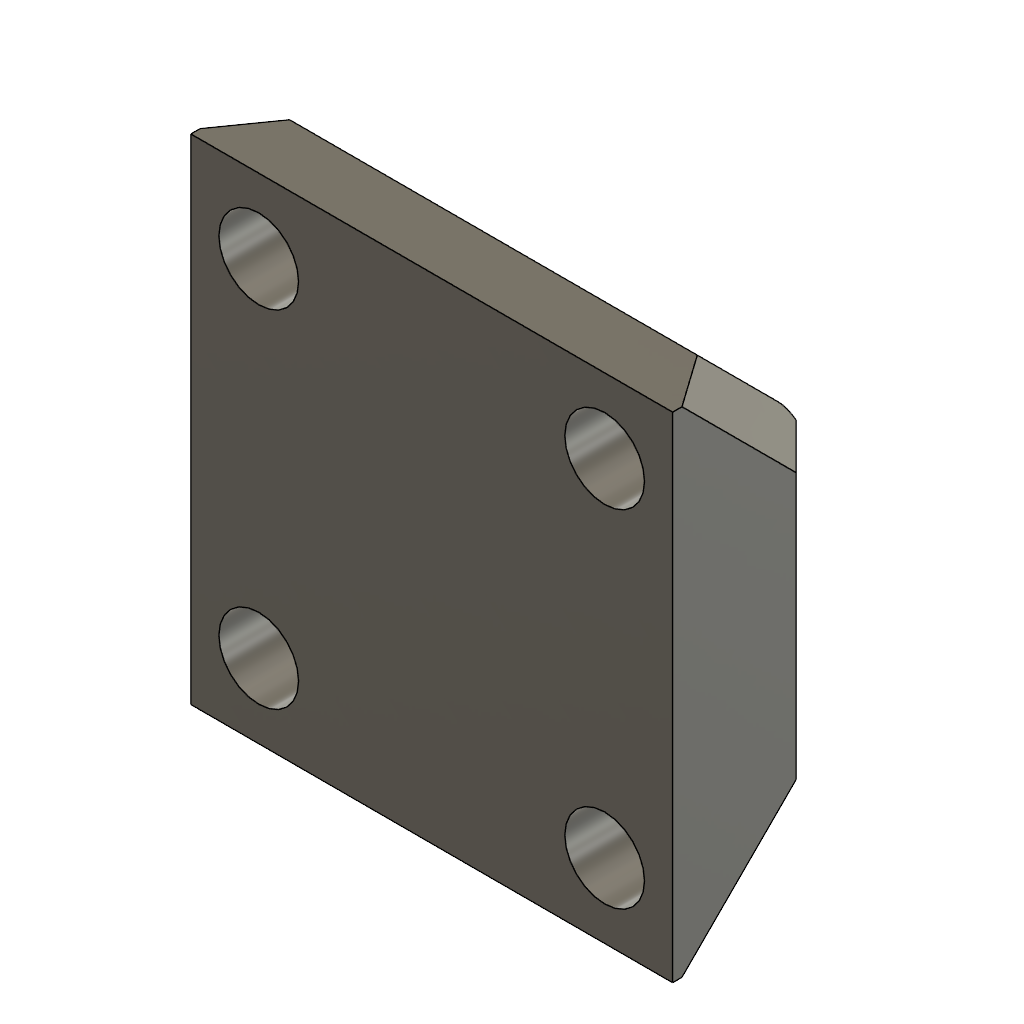
Gondola Sliding system (Autodesk Fusion 360 design; units mm, degrees)
part number: 2026-09-25-01-20-45-997
Autodesk Fusion 360 part; units mm, degrees
sketch "Sketch8" plane through (0, 0, 0) normal (0, 1, 0) x (1, 0, 0)
  line L0 (10, -20) -> (-29, -20)
  line L1 (-29, -20) -> (-29, -5)
  line L2 (-29, -5) -> (10, -5)
  line L3 (10, -5) -> (10, -20)
  dimension "d35" = 39
  dimension "d36" = 15
  constraint horizontal L0
  constraint vertical L1
  constraint horizontal L2
  constraint vertical L3
  measures "d35" distance of L0.start L0.end
  measures "d36" distance of L0.start L2.end
extrude "Extrude14" add sketch "Sketch8" along normal blind 40
sketch "Sketch10" plane through (0, 0, 20) normal (0, 0, 1) x (1, 0, 0)
  line L0 (-29, 0) -> (10, 0)
  line L1 (10, 0) -> (10, 40)
  line L2 (10, 40) -> (-29, 40)
  line L3 (-29, 40) -> (-29, 0)
  line L4 (1.275, 6) -> (-20.275, 6)
  line L5 (-23.5, 9.225) -> (-23.5, 30.775)
  line L6 (-20.275, 34) -> (1.275, 34)
  line L7 (4.5, 30.775) -> (4.5, 9.225)
  line L8 (2.2196, 8.2804) -> (-21.2196, 31.7196) construction
  line L9 (-21.2196, 8.2804) -> (2.2196, 31.7196) construction
  circle A0 centre (-23.5, 34) radius 3.225
  circle A1 centre (4.5, 34) radius 3.225
  circle A2 centre (4.5, 6) radius 3.225
  circle A3 centre (-23.5, 6) radius 3.225
  point P0 (-9.5, 20)
  dimension "d42" = 28
  dimension "d43" = 28
  dimension "d44" = 6.45
  dimension "d45" = 6.45
  dimension "d46" = 6.45
  dimension "d47" = 6.45
  constraint horizontal L4
  constraint perpendicular L4 L5
  constraint parallel L4 L6
  constraint parallel L5 L7
  constraint coincident L8 P0
  constraint coincident L9 P0
  constraint coincident A3 L5.start
  constraint coincident A3 L9.start
  constraint coincident A3 L4.end
  constraint coincident A2 L4.start
  constraint coincident A2 L8.start
  constraint coincident A2 L7.end
  constraint coincident A1 L7.start
  constraint coincident A1 L9.end
  constraint coincident A1 L6.end
  constraint coincident A0 L6.start
  constraint coincident A0 L8.end
  constraint coincident A0 L5.end
  measures "d42" distance of A0.centre A1.centre
  measures "d43" distance of A0.centre A3.centre
  measures "d44" diameter of A0
  measures "d45" diameter of A1
  measures "d46" diameter of A2
  measures "d47" diameter of A3
extrude "Extrude15" cut sketch "Sketch10" against normal blind 6.5 contours A2 | A3 | A1 | A0
chamfer "Chamfer1" distance 8 angle 45 2 edges at (-9.5, 40, 5) (-9.5, 0, 5) tangent chain off
chamfer "Chamfer2" distance 3 angle 45 6 edges at (-29, 36, 9) (-29, 20, 5) (-29, 4, 9) (10, 36, 9) (10, 20, 5) (10, 4, 9) tangent chain off
sketch "Sketch11" plane through (0, 0, 5) normal (0, 0, -1) x (-1, 0, 0)
  line L0 (-7, 32) -> (-7, 8)
  line L1 (-7, 8) -> (26, 8)
  line L2 (26, 8) -> (26, 32)
  line L3 (26, 32) -> (-7, 32)
  line L4 (9.5, 32) -> (9.5, 8)
  line L5 (-7, 32) -> (9.5, 32)
  circle A0 centre (-1, 20) radius 5.02
  circle A1 centre (20, 20) radius 5.02
  dimension "d52" = 10.04
  constraint midpoint L3 L4.start
  constraint midpoint L1 L4.end
  constraint coincident L0.start L3.end
  constraint symmetric L4 A0 A1
  measures "d52" diameter of A0
extrude "Extrude16" cut sketch "Sketch11" against normal blind 3 contours A0 | A1
extrude "Extrude17" cut 4 faces at (5.9059, 34.8722, 13.5) (4.282, 4.554, 13.5) (-23.2679, 7.0007, 13.5) (-22.5672, 33.9893, 13.5) along direction (0, 0, -1) blind 2
extrude "Extrude18" cut 1 faces at (-5.6214, 16.0645, 20) along direction (0, 0, -1) blind 2
fillet "Fillet1" radius 1 4 edges at (1.4932, 35.1662, 11.5) (-26.5068, 35.1662, 11.5) (-26.5068, 7.1662, 11.5) (1.4932, 7.1662, 11.5)
fillet "Fillet2" radius 0.3 2 edges at (5.6803, 21.8153, 5) (-15.3197, 21.8153, 5)
fillet "Fillet3" radius 5 2 edges at (-9.5, 32, 5) (-9.5, 8, 5)
